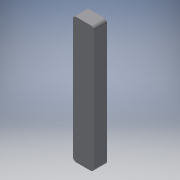
# Autodesk Inventor part: ConnectorRodBodies
Saved by Autodesk Inventor 2016 (Build 200138000, 138)
## iProperties
Created: 2017-03-11
Part Number: ConnectorRodBodies
Material: Generic
Document SubType Name: Modeling
Designer: Owner
Density: 1 g/cm^3
Appearance: Default
Author: Owner
Autodesk Inventor part; units mm, degrees
ref_plane "YZ Plane" through (0, 0, 0) normal (1, 0, 0) x (0, 1, 0)
ref_plane "XZ Plane" through (0, 0, 0) normal (0, 1, 0) x (-1, 0, 0)
ref_plane "XY Plane" through (0, 0, 0) normal (0, 0, 1) x (1, 0, 0)
sketch "Sketch1" plane through (0, 0, 0) normal (0, 0, 1) x (1, 0, 0)
  circle A0 centre (27.1, 34.2286) radius 4 projected
  circle A1 centre (27.1, 34.2286) radius 5 projected
  circle A2 centre (27.0777, 74.6286) radius 4 projected
  circle A3 centre (27.0777, 74.6286) radius 5 projected
  line L0 (32.0777, 76.0286) -> (34.0777, 76.0286)
  line L1 (34.0777, 76.0286) -> (34.0777, 78.0286)
  line L2 (29.7277, 29.2286) -> (27.7277, 29.2286)
  line L3 (27.7277, 29.2286) -> (27.7277, 27.2286)
  line L4 (27.7277, 27.2286) -> (34.0777, 27.2286)
  line L5 (34.0777, 27.2286) -> (34.0777, 78.0286)
  line L6 (34.0777, 78.0286) -> (27.7277, 78.0286)
  line L7 (27.7277, 78.0286) -> (27.7277, 27.2286)
  line L8 (20.0777, 74.6286) -> (27.7277, 412444959.5971)
  point P0 (0, 0)
  dimension "d0" = 2
  dimension "d1" = 2
  dimension "d2" = 2
  dimension "d3" = 2
  dimension "d8" = 50.8
  dimension "d14" = 6.35
  constraints: 17 end point, 3 horizontal, 3 parallel, 3 perpendicular, 1 vertical, 1 other
  measures "d0" distance of L0.start L0.end
  measures "d1" distance of L0.end L1.end
  measures "d2" distance of L2.start L2.end
  measures "d3" distance of L2.end L3.end
  measures "d8" distance of L1.end L4.end
  measures "d14" distance of L3.end L4.end
extrude "Extrusion2" add sketch "Sketch1" along normal blind 4 contours A0 L7 | A0 L7 A1 | L7 A3 L6 L1 L5 L4 L3 A1 | L7 A2 L6 A3 | L7 L6 A2 picked at (29.1356, 35.0943) picked at (31.6818, 33.5199) picked at (31.6654, 75.3088) picked at (28.0276, 73.2171)
sketch "Sketch2" plane through (0, 0, 4) normal (0, 0, 1) x (1, 0, 0)
  line L0 (34.0777, 27.2286) -> (34.0777, 78.0286) projected
  line L1 (34.0777, 27.2286) -> (34.0777, 39.9286)
  line L2 (27.7277, 78.0286) -> (27.7277, 27.2286) projected
  line L3 (34.0777, 39.9286) -> (27.7277, 39.9286)
  line L4 (27.7277, 39.9286) -> (27.7277, 27.2286)
  line L5 (27.7277, 27.2286) -> (34.0777, 27.2286)
  line L6 (34.0777, 27.2286) -> (34.0777, 39.9286)
  point P0 (0, 0)
  dimension "d15" = 12.7
  constraints: 10 end point, 2 parallel, 1 horizontal, 1 perpendicular, 1 point on line
  measures "d15" distance of L0.start L1.end
extrude "Extrusion3" cut sketch "Sketch2" against normal blind 25.4
fillet "Fillet2" radius 1 4 edges at (27.7277, 39.9286, 2) (34.0777, 39.9286, 2) (34.0777, 78.0286, 2) (27.7277, 78.0286, 2)
body "Solid2"
